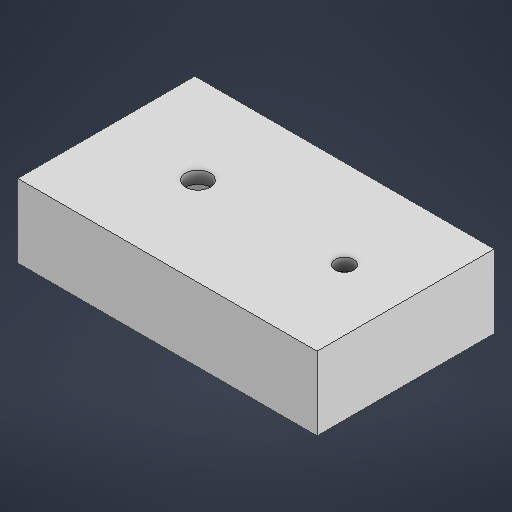
# Autodesk Inventor part: servoTest
Saved by Autodesk Inventor 2026 (Build 300175050, 175E)
## iProperties
Created: 2025-08-28
Part Number: servoTest
Material: Generic
Document SubType Name: Modeling
Designer: sidsi
Density: 1 g/cm^3
Appearance: Default
Author: sidsi
Autodesk Inventor part; units mm, degrees
ref_plane "YZ Plane" through (0, 0, 0) normal (1, 0, 0) x (0, 1, 0)
ref_plane "XZ Plane" through (0, 0, 0) normal (0, 1, 0) x (-1, 0, 0)
ref_plane "XY Plane" through (0, 0, 0) normal (0, 0, 1) x (1, 0, 0)
sketch "Sketch1" plane through (0, 0, 0) normal (0, 1, 0) x (-1, 0, 0)
  circle A0 centre (0, 0) radius 7.5
  line L0 (0, 3.75) -> (-24, 3.75)
  line L1 (-24, 3.75) -> (-24, -3.75)
  line L2 (-24, -3.75) -> (0, -3.75)
  line L3 (0, -3.75) -> (0, 3.75)
  circle A1 centre (-24, 0) radius 3.75
  line L4 (15, 14.5) -> (-34, 14.5)
  line L5 (-34, 14.5) -> (-34, -14.5)
  line L6 (-34, -14.5) -> (15, -14.5)
  line L7 (15, -14.5) -> (15, 14.5)
  point P0 (-6.4952, 3.75)
  point P1 (-6.4952, -3.75)
  dimension "d0" = 15
  dimension "d1" = 24
  dimension "d2" = 7.5
  dimension "d3" = 3.75
  dimension "d4" = 7
  dimension "d5" = 7
  dimension "d6" = 15
  dimension "d7" = 10
  constraints: 16 end point, 4 parallel, 2 centre point, 2 horizontal, 2 perpendicular, 1 coincident, 1 midpoint, 1 tangent
  measures "d0" diameter of A0
  measures "d1" distance of L2.end L1.end
  measures "d2" distance of L1.end L0.end
  measures "d3" distance from line of point (0, 0) L2
  measures "d4" distance edge to line of A0 L6
  measures "d5" distance edge to line of A0 L4
  measures "d6" distance from line of A0.centre L7
  measures "d7" distance from line of L5 A1.centre
extrude "Extrusion1" add sketch "Sketch1" along normal blind 10
fillet "Fillet1" radius 4 2 edges at (6.4952, 5, 3.75) (6.4952, 5, -3.75)
sketch "Sketch2" plane through (0, 10, 0) normal (0, 1, 0) x (1, 0, 0)
  line L0 (-15, 14.5) -> (-15, -14.5) projected
  line L1 (34, -14.5) -> (34, 14.5) projected
  line L2 (-15, -14.5) -> (34, -14.5)
  line L3 (34, -14.5) -> (34, 14.5)
  line L4 (34, 14.5) -> (-15, 14.5)
  line L5 (-15, 14.5) -> (-15, -14.5)
  point P0 (0, 0)
  constraints: 8 end point, 2 parallel, 1 horizontal, 1 perpendicular
extrude "Extrusion2" add sketch "Sketch2" along normal blind 2
sketch "Sketch3" plane through (0, 10, 0) normal (0, -1, 0) x (1, 0, 0)
  circle A0 centre (0, 0) radius 2
  arc A1 (24, -3.75) -> (24, 3.75) centre (24, 0) ccw projected
  circle A2 centre (24, 0) radius 1.5
  dimension "d13" = 4
  dimension "d14" = 3
  constraints: 2 centre point, 2 coincident
  measures "d13" diameter of A0
  measures "d14" diameter of A2
extrude "Extrusion3" cut sketch "Sketch3" against normal blind 2
body "Solid1"
